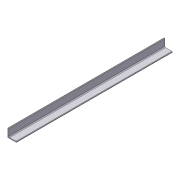
# Autodesk Inventor part: GE-12019-06
Saved by Autodesk Inventor 2012 (Build 160160000, 160)
## iProperties
Created: 2011-06-21
Part Number: GE-12019-06
Document SubType Name: Modeling
Designer: dfoster
Density: 2.71 g/cm^3
Material: Aluminum-6061
Mass: 2519.09 g
Surface Area: 3014.15 cm^2
Volume: 929.553 cm^3
Description: Angle, Bottom
Title: Angle, Bottom
Author: dfoster
Autodesk Inventor part; units mm, degrees
ref_plane "YZ Plane" through (0, 0, 0) normal (1, 0, 0) x (0, 1, 0)
ref_plane "XZ Plane" through (0, 0, 0) normal (0, 1, 0) x (-1, 0, 0)
ref_plane "XY Plane" through (0, 0, 0) normal (0, 0, 1) x (1, 0, 0)
sketch "Sketch1" plane through (0, 0, 0) normal (0, 0, 1) x (1, 0, 0)
  line L0 (0, 0) -> (0, 63.5)
  line L1 (0, 63.5) -> (3.175, 63.5)
  line L2 (6.35, 60.325) -> (6.35, 12.7)
  line L3 (12.7, 6.35) -> (60.325, 6.35)
  line L4 (63.5, 3.175) -> (63.5, 0)
  line L5 (63.5, 0) -> (0, 0)
  arc A0 (6.35, 12.7) -> (12.7, 6.35) centre (12.7, 12.7) ccw
  arc A1 (63.5, 3.175) -> (60.325, 6.35) centre (60.325, 3.175) ccw
  arc A2 (6.35, 60.325) -> (3.175, 63.5) centre (3.175, 60.325) ccw
  dimension "d0" = 63.5
  dimension "d1" = 6.35
  dimension "d2" = 6.35
  dimension "d3" = 3.175
  constraints: 12 end point, 6 point on circle, 6 tangent, 4 parallel, 3 centre point, 3 perpendicular, 1 equal radius, 1 vertical
  measures "d0" distance of L0.start L0.end
  measures "d1" distance between parallel lines of L2 L0
  measures "d2" radius of A0
  measures "d3" radius of A1
extrude "Extrusion1" add sketch "Sketch1" along normal blind 1181.1
body "Solid1"
